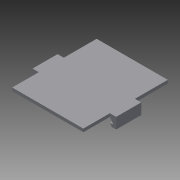
# Autodesk Inventor part: SkateBoxCover
Saved by Autodesk Inventor 2013 (Build 170138000, 138)
## iProperties
Created: 2015-10-02
Part Number: SkateBoxCover
Material: Generic
Document SubType Name: Modeling
Designer: A.Barredo
Density: 1 g/cm^3
Author: A.Barredo
Autodesk Inventor part; units mm, degrees
ref_plane "YZ Plane" through (0, 0, 0) normal (1, 0, 0) x (0, 1, 0)
ref_plane "XZ Plane" through (0, 0, 0) normal (0, 1, 0) x (-1, 0, 0)
ref_plane "XY Plane" through (0, 0, 0) normal (0, 0, 1) x (1, 0, 0)
sketch "Sketch1" plane through (0, 0, 0) normal (0, 0, 1) x (1, 0, 0)
  line L0 (-11.7277, 11.2879) -> (33.7723, 11.2879)
  line L1 (33.7723, 11.2879) -> (33.7723, -42.7121)
  line L2 (33.7723, -42.7121) -> (-11.7277, -42.7121)
  line L3 (-11.7277, -42.7121) -> (-11.7277, 11.2879)
  line L4 (-11.7277, -9.7121) -> (-15.7277, -9.7121)
  line L5 (-15.7277, -9.7121) -> (-15.7277, -23.7121)
  line L6 (-15.7277, -23.7121) -> (-11.7277, -23.7121)
  line L7 (-11.7277, -23.7121) -> (-11.7277, -9.7121)
  line L8 (33.7723, -9.7121) -> (37.7723, -9.7121)
  line L9 (37.7723, -9.7121) -> (37.7723, -23.7121)
  line L10 (37.7723, -23.7121) -> (33.7723, -23.7121)
  line L11 (33.7723, -23.7121) -> (33.7723, -9.7121)
  point P0 (0, 0)
  dimension "d0" = 45.5
  dimension "d1" = 54
  dimension "d2" = 4
  dimension "d3" = 14
  dimension "d4" = 21
  dimension "d5" = 4
  dimension "d6" = 14
  dimension "d7" = 21
  constraints: 24 end point, 6 parallel, 3 horizontal, 3 perpendicular, 2 point on line
  measures "d0" distance of L1.end L2.end
  measures "d1" distance of L0.end L1.end
  measures "d2" distance of L6.end L5.end
  measures "d3" distance of L4.end L5.end
  measures "d4" distance between parallel lines of L4 L0
  measures "d5" distance of L9.end L10.end
  measures "d6" distance of L8.end L9.end
  measures "d7" distance between parallel lines of L8 L0
extrude "Extrusion1" add sketch "Sketch1" along normal blind 2 contours L0 L1 L2 L3
sketch "Sketch2" plane through (0, 0, 2) normal (0, 0, 1) x (1, 0, 0)
  line L0 (-11.7277, 11.2879) -> (-11.7277, -42.7121) projected
  line L1 (33.7723, -42.7121) -> (33.7723, 11.2879) projected
  line L2 (33.7723, 11.2879) -> (-11.7277, 11.2879) projected
  line L3 (-11.7277, -9.7121) -> (-15.7277, -9.7121)
  line L4 (-15.7277, -9.7121) -> (-15.7277, -25.7121)
  line L5 (-15.7277, -25.7121) -> (-11.7277, -25.7121)
  line L6 (-11.7277, -25.7121) -> (-11.7277, -9.7121)
  line L7 (33.7723, -9.7121) -> (37.7723, -9.7121)
  line L8 (37.7723, -9.7121) -> (37.7723, -25.7121)
  line L9 (37.7723, -25.7121) -> (33.7723, -25.7121)
  line L10 (33.7723, -25.7121) -> (33.7723, -9.7121)
  point P0 (0, 0)
  dimension "d10" = 4
  dimension "d11" = 16
  dimension "d12" = 21
  dimension "d13" = 4
  constraints: 16 end point, 4 parallel, 2 horizontal, 2 perpendicular, 2 point on line
  measures "d10" distance of L5.end L4.end
  measures "d11" distance of L4.end L3.end
  measures "d12" distance between parallel lines of L3 L2
  measures "d13" distance of L8.end L9.end
extrude "Extrusion2" add sketch "Sketch2" against normal blind 7
sketch "Sketch3" plane through (33.7723, -9.7121, 2) normal (0, 1, 0) x (1, 0, 0)
  line L0 (4, 0) -> (4, 7) projected
  line L1 (0, 2) -> (0, 7) projected
  line L2 (0, 7) -> (0, 5.2)
  line L3 (0, 5.2) -> (2.1, 5.2)
  line L4 (2.1, 5.2) -> (0, 2)
  line L5 (0, 5.2) -> (0, 2)
  point P0 (-33.7723, 2)
  dimension "d16" = 1.8
  dimension "d17" = 2.1
  constraints: 8 end point, 2 perpendicular, 1 point on line
  measures "d16" distance of L1.end L2.end
  measures "d17" distance of L2.end L3.end
extrude "Extrusion3" cut sketch "Sketch3" against normal blind 24.75
sketch "Sketch4" plane through (-15.7277, -9.7121, 2) normal (0, 1, 0) x (1, 0, 0)
  line L0 (4, 2) -> (4, 7) projected
  line L1 (4, 7) -> (4, 5.2)
  line L2 (4, 5.2) -> (1.9, 5.2)
  line L3 (1.9, 5.2) -> (4, 2)
  point P0 (15.7277, 2)
  dimension "d20" = 1.8
  dimension "d21" = 2.1
  constraints: 6 end point, 1 perpendicular, 1 point on line
  measures "d20" distance of L0.end L1.end
  measures "d21" distance of L1.end L2.end
extrude "Extrusion4" cut sketch "Sketch4" against normal blind 176.5
sketch "Sketch5" plane through (-15.7277, -9.7121, 2) normal (0, 1, 0) x (1, 0, 0)
  line L0 (4, 5.2) -> (4, 7) projected
  line L1 (0, 7) -> (4, 7) projected
  line L2 (4, 2) -> (4, 0) projected
  line L3 (4, 2) -> (1.9, 5.2) projected
  line L4 (4, 5.2) -> (2.8188, 7)
  line L5 (4, 7) -> (4, 5.2)
  point P0 (15.7277, 2)
  constraints: 4 end point, 1 collinear, 1 parallel, 1 point on line
extrude "Extrusion5" cut sketch "Sketch5" against normal blind 3535.5
sketch "Sketch6" plane through (33.7723, -9.7121, 2) normal (0, 1, 0) x (1, 0, 0)
  line L0 (2.1, 5.2) -> (0, 2) projected
  line L1 (0, 7) -> (4, 7) projected
  line L2 (0, 5.2) -> (0, 7) projected
  line L3 (0, 5.2) -> (2.1, 5.2) projected
  line L4 (0, 5.2) -> (1.1813, 7)
  line L5 (0, 7) -> (0, 5.2)
  point P0 (-33.7723, 2)
  constraints: 4 end point, 1 parallel, 1 perpendicular, 1 point on line
extrude "Extrusion6" cut sketch "Sketch6" against normal blind 5309.5
body "Solid1"
